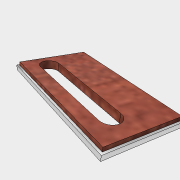
# Autodesk Inventor part: Shifter surround
Saved by Autodesk Inventor 2020.1 (Build 241239000, 239)
## iProperties
Created: 2019-09-13
Part Number: Shifter surround
Material: Generic
Document SubType Name: Modeling
Designer: thom_tremblay
Density: 1 g/cm^3
Appearance: Default
Author: thom_tremblay
Autodesk Inventor part; units mm, degrees
ref_plane "YZ Plane" through (0, 0, 0) normal (1, 0, 0) x (0, 1, 0)
ref_plane "XZ Plane" through (0, 0, 0) normal (0, 1, 0) x (-1, 0, 0)
ref_plane "XY Plane" through (0, 0, 0) normal (0, 0, 1) x (1, 0, 0)
sketch "Sketch1" plane through (0, 0, 0) normal (0, 0, 1) x (1, 0, 0)
  line L0 (0, 0) -> (76.2, 0)
  line L1 (76.2, 0) -> (76.2, 139.7)
  line L2 (76.2, 139.7) -> (0, 139.7)
  line L3 (0, 139.7) -> (0, 0)
  line L4 (15.6073, 25.4999) -> (15.6073, 120.9664)
  arc A0 (34.9423, 120.9664) -> (15.6073, 120.9664) centre (25.2748, 120.9664) ccw
  line L5 (34.9423, 120.9664) -> (34.9423, 25.4999)
  arc A1 (15.6073, 25.4999) -> (34.9423, 25.4999) centre (25.2748, 25.4999) ccw
  line L6 (2.202, 137.498) -> (73.998, 137.498)
  line L7 (73.998, 137.498) -> (73.998, 2.202)
  line L8 (73.998, 2.202) -> (2.202, 2.202)
  line L9 (2.202, 2.202) -> (2.202, 137.498)
  dimension "d0" = 76.2
  dimension "d1" = 139.7
  constraints: 20 end point, 4 parallel, 4 point on circle, 4 tangent, 2 centre point, 2 perpendicular, 2 vertical, 1 horizontal, 3 other
  measures "d0" distance of L2.end L1.end
  measures "d1" distance of L1.end L0.end
extrude "Extrusion1" add sketch "Sketch1" against normal blind 4.7625 contours L3 L2 L1 L0 | L6 L7 L8 L9
extrude "Extrusion2" add sketch "Sketch1" along normal blind 3.81 contours L6 L7 L8 L9
body "Solid1"
